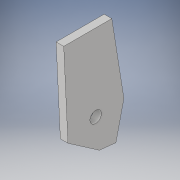
# Autodesk Inventor part: Handle Insert V1
Saved by Autodesk Inventor 2018 (Build 220112000, 112)
## iProperties
Created: 2017-09-20
Part Number: Handle Insert V1
Material: Generic
Document SubType Name: Modeling
Designer: Patrick
Density: 1 g/cm^3
Appearance: Default
Author: Patrick
Autodesk Inventor part; units mm, degrees
ref_plane "YZ Plane" through (0, 0, 0) normal (1, 0, 0) x (0, 1, 0)
ref_plane "XZ Plane" through (0, 0, 0) normal (0, 1, 0) x (-1, 0, 0)
ref_plane "XY Plane" through (0, 0, 0) normal (0, 0, 1) x (1, 0, 0)
sketch "Sketch1" plane through (0, 0, 0) normal (1, 0, 0) x (0, 1, 0)
  line L0 (0, 0) -> (0, -32.004)
  line L1 (6.1409, 0) -> (6.1409, -25.4) construction
  line L2 (0, -32.004) -> (-50.0461, -40.0442)
  line L3 (-50.0461, -40.0442) -> (-72.9333, -34.7254)
  line L4 (-72.9333, -34.7254) -> (-71.805, -23.7653)
  line L5 (-71.805, -23.7653) -> (-57.2991, -2.8123)
  line L6 (-57.2991, -2.8123) -> (0, 0)
  circle A0 centre (-51.308, -21.2399) radius 3.81
  dimension "d0" = 32.004
  dimension "d1" = 25.4
  dimension "d2" = 7.62
  dimension "d3" = 51.308
  constraints: 14 end point, 2 vertical, 1 centre point
  measures "d0" distance of L0.start L0.end
  measures "d1" distance of L1.start L1.end
  measures "d2" diameter of A0
  measures "d3" distance from line of L0 A0.centre
extrude "Extrusion1" add sketch "Sketch1" along normal blind 5.08
body "Solid1"
